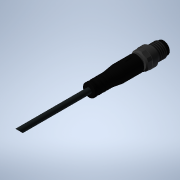
# Autodesk Inventor part: 8082090 SDBT-M8---(stecker)
Saved by Autodesk Inventor 2021 (Build 250183000, 183)
## iProperties
Created: 2025-06-25
Part Number: 8082090 SDBT-M8---(stecker)
Material: Generic
Catalog Web Link: www.cadenas.de
Description: SDBT-MSX_stecker-plug
Vendor: FESTO
Document SubType Name: Modeling
Designer: psAdmin
Manufacturer: FESTO
Mass: 2.18989 g
Surface Area: 16.9644 cm^2
Volume: 2.18989 cm^3
Density: 1 g/cm^3
Appearance: PSOLRGB-175-175-175
Category: PARTsolutions
Company: FESTO
Title: 8082090 SDBT-M8---(stecker)
Author: Cadenas PARTsolutions
Comments: plug
PSOL_IDENT_0: {$CADENAS_DATA/23d-libs/festo/parts/s/sdbt/parts/sdbt_msx_stecker.prj},206 {VTYP=3D},{NB=8082090 SDB
PSOL_IDENT_1: T-M8---(stecker)},{LINA=8082090 SDBT-M8---(stecker)},{NN=SDBT-MSX_stecker},{DATE=05.02.2025 08:34:15
PSOL_IDENT_2: },{GEOMDATE=05.02.2025 08:34:00},{VERSION=},{LINEID=10},{WBVAR=AT},{WBNUMERIC=}  {NB=8082090 SDBT-M8
PSOL_IDENT_3: ---(stecker)},{LINA=8082090 SDBT-M8---(stecker)},{KT=DUMMY},{TNR=8082090},{TYP=SDBT},{AT=M8},{D1=2.9
PSOL_IDENT_4: 00},{LL=40.000},{VER=1}
NB: 8082090 SDBT-M8---(stecker)
NN: SDBT-MSX_stecker
NT: plug
NBSYN: $TNR. $TYP.-$AT.---(stecker)
LINA: 8082090 SDBT-M8---(stecker)
CATALOG: Festo
TNR: 8082090
TYP: SDBT
AT: M8
D1: 2.9
LL: 40
SUPPLIER: FESTO
ARTICLENO: 8082090 SDBT-M8---(stecker)
BOMINFO: 8082090 SDBT-M8---(stecker)
CREATOR: CADENAS GmbH
Autodesk Inventor part; units mm, degrees
sketch "Sketch_14" plane through (0, 0, 0) normal (1, 0, 0) x (0, 1, 0)
  line L0 (0, -26.1) -> (0, 0)
  line L1 (0, 0) -> (3.2, 0)
  arc A0 (3.5, -0.3) -> (3.2, 0) centre (3.2, -0.3) ccw
  line L2 (3.5, -0.3) -> (3.5, -1.5)
  arc A1 (3.5, -1.5) -> (3.5, -3.5) centre (6.3284, -2.5) ccw
  line L3 (3.5, -3.5) -> (3.5, -4.5)
  arc A2 (3.5, -4.5) -> (3.5, -5.9) centre (5.4799, -5.2) ccw
  line L4 (3.5, -5.9) -> (3.5, -6.9)
  arc A3 (3.5, -6.9) -> (3.5, -7.9) centre (4.9142, -7.4) ccw
  line L5 (3.5, -7.9) -> (3.5, -8.9)
  arc A4 (3.5, -8.9) -> (3.5, -9.5) centre (4.3485, -9.2) ccw
  line L6 (3.5, -9.5) -> (3.5, -10.5)
  line L7 (3.5, -10.5) -> (4.25, -15.9)
  line L8 (4.25, -15.9) -> (4.25, -26.1)
  line L9 (4.25, -26.1) -> (0, -26.1)
  line L10 (0, -26.1) -> (0, 0)
  constraints: 22 end point, 10 point on circle, 5 centre point
revolve "Revolution1" add sketch "Sketch_14" angle 360 about axis through (0, 0, -26.1) along (0, 0, -1)
sketch "Sketch_13" plane through (0, 0, -21) normal (0, 0, 1) x (1, 0, 0)
  line L0 (5, -1.85) -> (-5, -1.85)
  circle A0 centre (0, 3.9556) radius 0.6944
  constraints: 2 end point, 1 centre point
revolve "Revolution2" add sketch "Sketch_13" angle 80 mid plane about axis through (5, -1.85, -21) along (-1, 0, 0)
sketch "Sketch_15" plane through (0, 0, -21) normal (0, 0, 1) x (1, 0, 0)
  line L0 (-5, 1.85) -> (5, 1.85)
  circle A0 centre (0, -3.9556) radius 0.6944
  constraints: 2 end point, 1 centre point
revolve "Revolution3" add sketch "Sketch_15" angle 80 mid plane about axis through (-5, 1.85, -21) along (1, 0, 0)
sketch "Sketch_7" plane through (0, 0, 0) normal (1, 0, 0) x (0, 1, 0)
  line L0 (0, -41.1) -> (0, -26.1)
  line L1 (0, -26.1) -> (2.95, -26.1)
  line L2 (2.95, -26.1) -> (2.95, -28.6)
  line L3 (2.95, -28.6) -> (3.15, -28.6)
  line L4 (3.15, -28.6) -> (3.15, -39.35)
  line L5 (3.15, -39.35) -> (3.45, -39.35)
  line L6 (3.45, -39.35) -> (3.45, -41.1)
  line L7 (3.45, -41.1) -> (2.9, -41.1)
  line L8 (2.9, -41.1) -> (2.9, -40.8)
  line L9 (2.9, -40.8) -> (0, -40.8)
  line L10 (0, -40.8) -> (0, -26.1)
  constraints: 22 end point
revolve "Revolution4" add sketch "Sketch_7" angle 360 about axis through (0, 0, -41.1) along (0, 0, -1)
sketch "Sketch_8" plane through (0, 0, 0) normal (1, 0, 0) x (0, 1, 0)
  line L0 (0, -39.35) -> (0, -27.45)
  line L1 (0, -27.45) -> (4.05, -27.45)
  line L2 (4.05, -27.45) -> (4.775, -28.175)
  line L3 (4.775, -28.175) -> (4.775, -30.45)
  line L4 (4.775, -30.45) -> (4.975, -30.45)
  line L5 (4.975, -30.45) -> (4.975, -33.25)
  line L6 (4.975, -33.25) -> (4.2, -33.25)
  arc A0 (4.2, -33.25) -> (4, -33.45) centre (4.2, -33.45) ccw
  line L7 (4, -33.45) -> (4, -39.1379)
  line L8 (4, -39.1379) -> (3.7879, -39.35)
  line L9 (3.7879, -39.35) -> (0, -39.35)
  line L10 (0, -39.35) -> (0, -27.45)
  constraints: 22 end point, 2 point on circle, 1 centre point
revolve "Revolution5" add sketch "Sketch_8" angle 360 about axis through (0, 0, -39.35) along (0, 0, -1)
thread "Thread1" size "M8x1" class "6g" standard "ISO Metric profile" length 4.2879
sketch "Sketch_10" plane through (0, 0, -27.45) normal (0, 0, 1) x (1, 0, 0)
  line L0 (-8, -8) -> (8, -8)
  line L1 (8, -8) -> (8, 8)
  line L2 (8, 8) -> (-8, 8)
  line L3 (-8, 8) -> (-8, -8)
  line L4 (-4.5, -2.5981) -> (0, -5.1962)
  line L5 (0, -5.1962) -> (4.5, -2.5981)
  line L6 (4.5, -2.5981) -> (4.5, 2.5981)
  line L7 (4.5, 2.5981) -> (0, 5.1962)
  line L8 (0, 5.1962) -> (-4.5, 2.5981)
  line L9 (-4.5, 2.5981) -> (-4.5, -2.5981)
  constraints: 20 end point
extrude "Extrusion1" cut sketch "Sketch_10" against normal blind 3
sketch "Sketch_9" plane through (0, 0, -40.8) normal (0, 0, 1) x (1, 0, 0)
  circle A0 centre (0, 0) radius 2.9
  circle A1 centre (1.75, 0) radius 0.5
  circle A2 centre (0, -1.75) radius 0.5
  circle A3 centre (-1.75, 0) radius 0.5
  constraints: 4 centre point
extrude "Extrusion2" cut sketch "Sketch_9" along normal blind 4.7
sketch "Sketch_3" plane through (0, 0, 0) normal (1, 0, 0) x (0, 1, 0)
  line L0 (0, 0) -> (0, 40)
  line L1 (0, 40) -> (1.45, 40)
  line L2 (1.45, 40) -> (1.45, 0)
  line L3 (1.45, 0) -> (0, 0)
  line L4 (0, 0) -> (0, 40)
  constraints: 10 end point
revolve "Revolution6" add sketch "Sketch_3" angle 360 about axis through (0, 0, 0) along (0, 0, -1)
sketch "Sketch_4" plane through (0, 0, 0) normal (1, 0, 0) x (0, 1, 0)
  line L0 (1.45, 40) -> (-1.45, 40)
  line L1 (-1.45, 40) -> (-1.45, 37.1)
  line L2 (-1.45, 37.1) -> (1.45, 40)
  constraints: 6 end point
extrude "Extrusion3" cut sketch "Sketch_4" along normal mid plane 12
ref_plane "ANBAU_XY" through (0, 0, 40) normal (0, 0, 1) x (1, 0, 0)
ref_plane "ANBAU_YZ" through (0, 0, 40) normal (1, 0, 0) x (0, 1, 0)
ref_plane "ANBAU_ZX" through (0, 0, 40) normal (0, 1, 0) x (0, 0, 1)
ref_plane "ASCF1_XY" through (0, 0, 7) normal (0, 0, 1) x (1, 0, 0)
ref_plane "ASCF1_YZ" through (0, 0, 7) normal (1, 0, 0) x (0, 1, 0)
ref_plane "ASCF1_ZX" through (0, 0, 7) normal (0, 1, 0) x (0, 0, 1)
ref_plane "CONN_XY" through (0, 0, 0) normal (0, 0, -1) x (1, 0, 0)
ref_plane "CONN_YZ" through (0, 0, 0) normal (1, 0, 0) x (0, -1, 0)
ref_plane "CONN_ZX" through (0, 0, 0) normal (0, -1, 0) x (0, 0, -1)
ref_plane "FDT_CONCAB_XY" through (0, 0, -36.1) normal (0, 0, -1) x (0, -1, 0)
ref_plane "FDT_CONCAB_YZ" through (0, 0, -36.1) normal (0, -1, 0) x (-1, 0, 0)
ref_plane "FDT_CONCAB_ZX" through (0, 0, -36.1) normal (-1, 0, 0) x (0, 0, -1)
body "Solid1"
